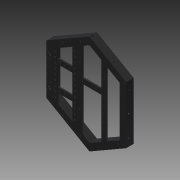
# Autodesk Inventor part: TSOP Array
Saved by Autodesk Inventor 2015 (Build 190159000, 159)
## iProperties
Created: 2016-02-25
Part Number: TSOP Array
Material: ABS Plastic
Document SubType Name: Modeling
Designer: James Yelland
Density: 1.06 g/cm^3
Appearance: Smooth - White
Mass: 118.644 g
Surface Area: 498.11 cm^2
Volume: 111.928 cm^3
Author: James Yelland
Autodesk Inventor part; units mm, degrees
ref_plane "YZ Plane" through (0, 0, 0) normal (1, 0, 0) x (0, 1, 0)
ref_plane "XZ Plane" through (0, 0, 0) normal (0, 1, 0) x (-1, 0, 0)
ref_plane "XY Plane" through (0, 0, 0) normal (0, 0, 1) x (1, 0, 0)
sketch "Sketch1" plane through (0, 0, 0) normal (0, 1, 0) x (-1, 0, 0)
  line L0 (0, 100) -> (86.6025, 50)
  line L1 (86.6025, 50) -> (86.6025, -50)
  line L2 (86.6025, -50) -> (0, -100)
  line L3 (0, 85) -> (73.6122, 42.5)
  line L4 (73.6122, 42.5) -> (73.6122, -42.5)
  line L5 (73.6122, -42.5) -> (0, -85)
  circle A0 centre (-69.3774, 54.1653) radius 1.6
  line L6 (-60.6222, 0) -> (-60.6222, -49.9998)
  line L7 (-60.6222, 0) -> (-60.6222, 49.9998)
  line L8 (0, -85) -> (-60.6222, -49.9998)
  line L9 (-60.6222, 49.9998) -> (0, 85)
  line L10 (-73.6122, -57.5) -> (-73.6122, 57.5)
  line L11 (0, 100) -> (-73.6122, 57.5)
  line L12 (-73.6122, -57.5) -> (0, -100)
  circle A1 centre (-69.3774, -54.1745) radius 1.6
  line L13 (-68.5014, -5.4) -> (-63.7014, -5.4)
  line L14 (-63.7014, -5.4) -> (-63.7014, 5.4)
  line L15 (-63.7014, 5.4) -> (-68.5014, 5.4)
  arc A2 (-68.5014, 2.5807) -> (-68.5014, -2.5807) centre (-67.5514, 0) ccw
  line L16 (-68.5014, -5.4) -> (-68.5014, -2.5807)
  line L17 (-68.5014, 2.5807) -> (-68.5014, 5.4)
  line L18 (-70.3014, 0) -> (-67.5514, 0)
  line L19 (-67.5514, 0) -> (-73.5514, 0)
  line L20 (-66.5387, -44.6515) -> (-62.3818, -42.2515)
  line L21 (-62.3818, -42.2515) -> (-67.7818, -32.8985)
  line L22 (-67.7818, -32.8985) -> (-71.9387, -35.2985)
  arc A3 (-70.5291, -37.7401) -> (-67.9484, -42.2099) centre (-68.416, -39.5) ccw
  line L23 (-66.5387, -44.6515) -> (-67.9484, -42.2099)
  line L24 (-70.5291, -37.7401) -> (-71.9387, -35.2985)
  line L25 (-70.7976, -40.875) -> (-68.416, -39.5)
  line L26 (-68.416, -39.5) -> (-73.6122, -42.5)
  line L27 (-36.0997, -73.3266) -> (-33.6997, -69.1696)
  line L28 (-33.6997, -69.1696) -> (-43.0528, -63.7696)
  line L29 (-43.0528, -63.7696) -> (-45.4528, -67.9266)
  arc A4 (-43.0112, -69.3362) -> (-38.5413, -71.9169) centre (-40.3013, -69.8038) ccw
  line L30 (-36.0997, -73.3266) -> (-38.5413, -71.9169)
  line L31 (-43.0112, -69.3362) -> (-45.4528, -67.9266)
  line L32 (-41.6763, -72.1854) -> (-40.3013, -69.8038)
  line L33 (-40.3013, -69.8038) -> (-43.3013, -75)
  line L34 (5.4, -94.95) -> (5.4, -90.15)
  line L35 (5.4, -90.15) -> (-5.4, -90.15)
  line L36 (-5.4, -90.15) -> (-5.4, -94.95)
  arc A5 (-2.5807, -94.95) -> (2.5807, -94.95) centre (0, -94) ccw
  line L37 (5.4, -94.95) -> (2.5807, -94.95)
  line L38 (-2.5807, -94.95) -> (-5.4, -94.95)
  line L39 (0, -96.75) -> (0, -94)
  line L40 (0, -94) -> (0, -100)
  line L41 (45.4528, -67.9266) -> (43.0528, -63.7696)
  line L42 (43.0528, -63.7696) -> (33.6997, -69.1696)
  line L43 (33.6997, -69.1696) -> (36.0997, -73.3266)
  arc A6 (38.5413, -71.9169) -> (43.0112, -69.3362) centre (40.3013, -69.8038) ccw
  line L44 (45.4528, -67.9266) -> (43.0112, -69.3362)
  line L45 (38.5413, -71.9169) -> (36.0997, -73.3266)
  line L46 (41.6763, -72.1854) -> (40.3013, -69.8038)
  line L47 (40.3013, -69.8038) -> (43.3013, -75)
  line L48 (84.9291, -42.7985) -> (80.7722, -40.3985)
  line L49 (80.7722, -40.3985) -> (75.3722, -49.7515)
  line L50 (75.3722, -49.7515) -> (79.5291, -52.1515)
  arc A7 (80.9388, -49.7099) -> (83.5195, -45.2401) centre (81.4064, -47) ccw
  line L51 (84.9291, -42.7985) -> (83.5195, -45.2401)
  line L52 (80.9388, -49.7099) -> (79.5291, -52.1515)
  line L53 (83.788, -48.375) -> (81.4064, -47)
  line L54 (81.4064, -47) -> (86.6025, -50)
  line L55 (81.5525, 5.4) -> (76.7525, 5.4)
  line L56 (76.7525, 5.4) -> (76.7525, -5.4)
  line L57 (76.7525, -5.4) -> (81.5525, -5.4)
  arc A8 (81.5525, -2.5807) -> (81.5525, 2.5807) centre (80.6025, 0) ccw
  line L58 (81.5525, 5.4) -> (81.5525, 2.5807)
  line L59 (81.5525, -2.5807) -> (81.5525, -5.4)
  line L60 (83.3525, 0) -> (80.6025, 0)
  line L61 (80.6025, 0) -> (86.6025, 0)
  line L62 (79.5291, 52.1515) -> (75.3722, 49.7515)
  line L63 (75.3722, 49.7515) -> (80.7722, 40.3985)
  line L64 (80.7722, 40.3985) -> (84.9291, 42.7985)
  arc A9 (83.5195, 45.2401) -> (80.9388, 49.7099) centre (81.4064, 47) ccw
  line L65 (79.5291, 52.1515) -> (80.9388, 49.7099)
  line L66 (83.5195, 45.2401) -> (84.9291, 42.7985)
  line L67 (83.788, 48.375) -> (81.4064, 47)
  line L68 (81.4064, 47) -> (86.6025, 50)
  line L69 (36.0997, 73.3266) -> (33.6997, 69.1696)
  line L70 (33.6997, 69.1696) -> (43.0528, 63.7696)
  line L71 (43.0528, 63.7696) -> (45.4528, 67.9266)
  arc A10 (43.0112, 69.3362) -> (38.5413, 71.9169) centre (40.3013, 69.8038) ccw
  line L72 (36.0997, 73.3266) -> (38.5413, 71.9169)
  line L73 (43.0112, 69.3362) -> (45.4528, 67.9266)
  line L74 (41.6763, 72.1854) -> (40.3013, 69.8038)
  line L75 (40.3013, 69.8038) -> (43.3013, 75)
  line L76 (-5.4, 94.95) -> (-5.4, 90.15)
  line L77 (-5.4, 90.15) -> (5.4, 90.15)
  line L78 (5.4, 90.15) -> (5.4, 94.95)
  arc A11 (2.5807, 94.95) -> (-2.5807, 94.95) centre (0, 94) ccw
  line L79 (-5.4, 94.95) -> (-2.5807, 94.95)
  line L80 (2.5807, 94.95) -> (5.4, 94.95)
  line L81 (0, 96.75) -> (0, 94)
  line L82 (0, 94) -> (0, 100)
  line L83 (-45.4528, 67.9266) -> (-43.0528, 63.7696)
  line L84 (-43.0528, 63.7696) -> (-33.6997, 69.1696)
  line L85 (-33.6997, 69.1696) -> (-36.0997, 73.3266)
  arc A12 (-38.5413, 71.9169) -> (-43.0112, 69.3362) centre (-40.3013, 69.8038) ccw
  line L86 (-45.4528, 67.9266) -> (-43.0112, 69.3362)
  line L87 (-38.5413, 71.9169) -> (-36.0997, 73.3266)
  line L88 (-41.6763, 72.1854) -> (-40.3013, 69.8038)
  line L89 (-40.3013, 69.8038) -> (-43.3013, 75)
  line L90 (-71.9387, 35.2985) -> (-67.7818, 32.8985)
  line L91 (-67.7818, 32.8985) -> (-62.3818, 42.2515)
  line L92 (-62.3818, 42.2515) -> (-66.5387, 44.6515)
  arc A13 (-67.9484, 42.2099) -> (-70.5291, 37.7401) centre (-68.416, 39.5) ccw
  line L93 (-71.9387, 35.2985) -> (-70.5291, 37.7401)
  line L94 (-67.9484, 42.2099) -> (-66.5387, 44.6515)
  line L95 (-70.7976, 40.875) -> (-68.416, 39.5)
  line L96 (-68.416, 39.5) -> (-73.6122, 42.5)
  dimension "d5" = 360
  dimension "d293" = 360
  dimension "d153" = 3.2
  dimension "d154" = 3.2
  dimension "d274" = 5.4
  dimension "d275" = 4.8
  dimension "d276" = 10.8
  dimension "d284" = 2.75
  dimension "d285" = 1.8
  dimension "d286" = 6
  constraints: 194 end point, 25 point on circle, 14 centre point, 1 point on line
  measures "d153" diameter of A1
  measures "d154" diameter of A0
  measures "d274" distance from line of L13 L18.end
  measures "d275" distance of L13.start L13.end
  measures "d276" distance of L13.end L14.end
  measures "d284" radius of A2
  measures "d285" horizontal distance of L18.start L13.start
  measures "d286" distance of L18.end L19.end
extrude "Extrusion1" add sketch "Sketch1" along normal blind 15 contours L0 L1 L2 L12 L10 L11 | A0 | A1
sketch "Sketch5" plane through (0, 15, 0) normal (0, 1, 0) x (1, 0, 0)
  circle A0 centre (-53.7917, 63.1699) radius 1.6
  circle A1 centre (-53.7917, -63.1699) radius 1.6
  line L0 (-73.6122, -42.5) -> (-73.6122, 42.5) projected
  line L1 (-73.6122, 42.5) -> (0, 85) projected
  line L2 (0, -85) -> (-73.6122, -42.5) projected
  line L3 (-86.6025, -50) -> (0, -100) projected
  line L4 (0, 100) -> (-86.6025, 50) projected
  line L5 (-86.6025, 50) -> (-86.6025, -50) projected
  circle A2 centre (69.3801, -54.1699) radius 1.6
  circle A3 centre (69.3801, 54.1699) radius 1.6
  line L6 (60.6222, -49.9998) -> (0, -85) projected
  line L7 (0, 85) -> (60.6222, 49.9998) projected
  line L8 (60.6222, 49.9998) -> (60.6222, -49.9998) projected
  line L9 (0, -100) -> (73.6122, -57.5) projected
  line L10 (73.6122, -57.5) -> (73.6122, 57.5) projected
  line L11 (73.6122, 57.5) -> (0, 100) projected
  point P0 (0, 0)
  dimension "d31" = 3.2
  dimension "d34" = 3.2
  dimension "d155" = 3.2
  dimension "d156" = 3.2
  constraints: 4 centre point
  measures "d31" diameter of A0
  measures "d34" diameter of A1
  measures "d155" diameter of A2
  measures "d156" diameter of A3
extrude "Extrusion5" cut sketch "Sketch5" against normal through all contours A0 | A1 | A2 | A3
sketch "Sketch6" plane through (0, 0, 0) normal (0, -1, 0) x (1, 0, 0)
  circle A0 centre (-29.6096, -40) radius 1.6
  circle A1 centre (-19.6096, 46.1471) radius 1.6
  circle A2 centre (28.6122, 39.8205) radius 1.6
  circle A3 centre (28.6122, -35.0619) radius 1.6
  circle A4 centre (13.3775, 15.699) radius 1.6
  circle A5 centre (-14.5314, 15.699) radius 1.6
  line L0 (-14.531, 20.699) -> (-14.6092, 20.699)
  line L1 (-14.6092, 20.699) -> (23.6131, 20.699)
  line L2 (23.6126, 10.699) -> (-14.6092, 10.699)
  line L3 (-73.6122, -42.5) -> (-63.6122, -48.2735)
  line L4 (-73.6122, -42.5) -> (-73.6122, 42.5)
  line L5 (-63.6122, 48.2735) -> (-73.6122, 42.5)
  circle A6 centre (-29.6096, 50) radius 1.6
  circle A7 centre (-29.6096, -50) radius 1.6
  line L6 (-63.6122, -20) -> (-34.6092, -20)
  line L7 (-63.6122, -30) -> (-34.6092, -30)
  line L8 (-63.6122, 20) -> (-34.6092, 20)
  line L9 (-34.6092, 30) -> (-63.6122, 30)
  line L10 (-63.6122, 30) -> (-63.6122, 48.2735)
  line L11 (-63.6122, -30) -> (-63.6122, -48.2735)
  line L12 (-34.6092, -20) -> (-34.6092, 20)
  circle A8 centre (-29.6096, -30) radius 1.6
  circle A9 centre (-29.6096, -20) radius 1.6
  circle A10 centre (-29.6096, -10) radius 1.6
  circle A11 centre (-29.6096, 0) radius 1.6
  circle A12 centre (-29.6096, 10) radius 1.6
  circle A13 centre (-29.6096, 20) radius 1.6
  circle A14 centre (-29.6096, 30) radius 1.6
  circle A15 centre (-29.6096, 40) radius 1.6
  circle A16 centre (-29.6096, 60) radius 1.6
  circle A17 centre (-29.6096, -60) radius 1.6
  circle A18 centre (-39.1109, 25) radius 1.6
  circle A19 centre (-49.1109, 25) radius 1.6
  circle A20 centre (-59.1109, 25) radius 1.6
  circle A21 centre (-39.1109, -25) radius 1.6
  circle A22 centre (-49.1109, -25) radius 1.6
  circle A23 centre (-59.1109, -25) radius 1.6
  circle A24 centre (-68.6122, -40) radius 1.6
  circle A25 centre (-68.6122, -30) radius 1.6
  circle A26 centre (-68.6122, -20) radius 1.6
  circle A27 centre (-68.6122, -10) radius 1.6
  circle A28 centre (-68.6122, 0) radius 1.6
  circle A29 centre (-68.6122, 10) radius 1.6
  circle A30 centre (-68.6122, 20) radius 1.6
  circle A31 centre (-68.6122, 30) radius 1.6
  circle A32 centre (-68.6122, 40) radius 1.6
  circle A33 centre (-19.6096, -36.3314) radius 1.6
  line L13 (-19.6096, 10) -> (-29.6096, 10)
  line L14 (23.6126, -71.3672) -> (33.6126, -65.5937)
  line L15 (23.6131, 71.367) -> (33.6126, 65.5937)
  line L16 (-34.6092, 65.0184) -> (-14.6092, 76.5654)
  line L17 (-14.6092, 10.699) -> (-14.6092, -76.5654)
  line L18 (-14.6092, -76.5654) -> (-34.6092, -65.0184)
  line L19 (-14.6092, 20.699) -> (-14.6092, 76.5654)
  line L20 (23.6131, 20.699) -> (23.6131, 71.367)
  line L21 (23.6126, -71.3672) -> (23.6126, 10.699)
  line L22 (33.6126, -65.5937) -> (33.6126, 65.5937)
  line L23 (-34.6092, 30) -> (-34.6092, 65.0184)
  line L24 (-34.6092, -65.0184) -> (-34.6092, -30)
  line L25 (-63.6122, -20) -> (-63.6122, 20)
  line L26 (-73.6122, -42.5) -> (-73.6122, 42.5)
  point P0 (0, -13.7917)
  dimension "d168" = 3.2
  dimension "d169" = 3.2
  dimension "d170" = 3.2
  dimension "d171" = 3.2
  dimension "d209" = 3.2
  dimension "d222" = 10
  constraints: 54 end point, 34 centre point, 12 vertical, 1 collinear, 1 horizontal, 1 point on line
  measures "d168" diameter of A5
  measures "d169" diameter of A4
  measures "d170" diameter of A2
  measures "d171" diameter of A3
  measures "d209" diameter of A33
  measures "d222" distance of L13.start L13.end
extrude "Extrusion6" add sketch "Sketch6" against normal blind 3
sketch "Sketch7" plane through (0, 15, 0) normal (0, 1, 0) x (1, 0, 0)
  circle A0 centre (69.3801, 54.1699) radius 1.6 projected
  circle A1 centre (-53.7917, 63.1699) radius 1.6 projected
  circle A2 centre (-53.7917, -63.1699) radius 1.6 projected
  circle A3 centre (69.3801, -54.1699) radius 1.6 projected
  line L0 (-73.6122, -42.5) -> (-73.6122, 42.5) projected
  line L1 (-73.6122, 42.5) -> (0, 85) projected
  line L2 (0, -85) -> (-73.6122, -42.5) projected
  line L3 (-86.6025, -50) -> (0, -100) projected
  line L4 (0, 100) -> (-86.6025, 50) projected
  line L5 (-86.6025, 50) -> (-86.6025, -50) projected
  circle A4 centre (-80.1075, -20) radius 1.6
  circle A5 centre (-80.1075, 20) radius 1.6
  line L6 (60.6222, -49.9998) -> (0, -85) projected
  line L7 (0, 85) -> (60.6222, 49.9998) projected
  line L8 (60.6222, 49.9998) -> (60.6222, -49.9998) projected
  line L9 (0, -100) -> (73.6122, -57.5) projected
  line L10 (73.6122, -57.5) -> (73.6122, 57.5) projected
  line L11 (73.6122, 57.5) -> (0, 100) projected
  line L12 (0, 100) -> (73.6122, 57.5) projected
  circle A6 centre (-18.3996, -81.8767) radius 1.6
  circle A7 centre (57.3685, -59.3781) radius 1.6
  line L13 (73.6122, -57.5) -> (73.6122, 57.5) projected
  circle A8 centre (-18.4029, 81.8748) radius 1.6
  circle A9 centre (57.3685, 59.3781) radius 1.6
  line L14 (0, 100) -> (-86.6025, 50) projected
  line L15 (-15.1376, -76.2603) -> (-18.3996, -81.8767)
  line L16 (-73.6122, 42.5) -> (0, 85) projected
  line L17 (-15.1554, 76.25) -> (-18.4029, 81.8748)
  line L18 (0, 85) -> (60.6222, 49.9998) projected
  line L19 (54.121, 53.7532) -> (57.3685, 59.3781)
  line L20 (54.121, -53.7532) -> (57.3685, -59.3781)
  point P0 (0, 0)
  dimension "d135" = 6.495
  dimension "d136" = 6.495
  dimension "d138" = 6.495
  dimension "d139" = 6.495
  dimension "d157" = 3.2
  dimension "d158" = 3.2
  dimension "d159" = 3.2
  dimension "d160" = 3.2
  dimension "d161" = 3.2
  dimension "d162" = 3.2
  constraints: 8 end point, 6 centre point, 4 point on line
  measures "d135" distance of L15.start L15.end
  measures "d136" distance of L17.start L17.end
  measures "d138" distance of L19.start L19.end
  measures "d139" distance of L20.start L20.end
  measures "d157" diameter of A6
  measures "d158" diameter of A4
  measures "d159" diameter of A5
  measures "d160" diameter of A8
  measures "d161" diameter of A9
  measures "d162" diameter of A7
extrude "Extrusion7" cut sketch "Sketch7" against normal through all contours A4 | A5 | A6 | A7 | A8 | A9
sketch "Sketch10" plane through (0, 15, 0) normal (0, 1, 0) x (1, 0, 0)
  circle A0 centre (69.3801, 54.1699) radius 1.6 projected
  circle A1 centre (-53.7917, 63.1699) radius 1.6 projected
  circle A2 centre (-53.7917, -63.1699) radius 1.6 projected
  circle A3 centre (69.3801, -54.1699) radius 1.6 projected
  line L0 (60.6222, -49.9998) -> (0, -85) projected
  line L1 (0, -85) -> (-73.6122, -42.5) projected
  line L2 (-73.6122, -42.5) -> (-73.6122, 42.5) projected
  line L3 (-73.6122, 42.5) -> (0, 85) projected
  line L4 (0, 85) -> (60.6222, 49.9998) projected
  line L5 (60.6222, 49.9998) -> (60.6222, -49.9998) projected
  line L6 (0, -100) -> (73.6122, -57.5) projected
  line L7 (73.6122, -57.5) -> (73.6122, 57.5) projected
  line L8 (73.6122, 57.5) -> (0, 100) projected
  line L9 (0, 100) -> (-86.6025, 50) projected
  line L10 (-86.6025, 50) -> (-86.6025, -50) projected
  line L11 (-86.6025, -50) -> (0, -100) projected
  circle A4 centre (-80.1075, 30) radius 3
  circle A5 centre (-80.1075, -30) radius 3
  point P0 (0, 0)
  dimension "d142" = 6
  dimension "d144" = 6
  constraints: 2 centre point
  measures "d142" diameter of A4
  measures "d144" diameter of A5
extrude "Extrusion10" cut sketch "Sketch10" against normal through all contours A4 | A5
sketch "Sketch13" plane through (60.6222, 0, 49.9998) normal (-1, 0, 0) x (0, 0, 1)
  circle A0 centre (-71.9998, 3) radius 1.4
  circle A1 centre (-27.9998, 3) radius 1.4
  circle A2 centre (-39.5858, 3.175) radius 1.4
  circle A3 centre (-60.4138, 3.175) radius 1.4
  dimension "d213" = 2.8
  dimension "d217" = 2.8
  dimension "d218" = 2.8
  constraints: 4 centre point
  measures "d213" diameter of A0
  measures "d217" diameter of A2
  measures "d218" diameter of A3
extrude "Extrusion12" cut sketch "Sketch13" against normal blind 10
sketch "Sketch20" plane through (0, 0, 0) normal (0, -1, 0) x (1, 0, 0)
  circle A0 centre (-80.1075, -30) radius 3 projected
  circle A1 centre (-80.1075, 30) radius 3 projected
  circle A2 centre (-18.4029, -81.8748) radius 1.6 projected
  circle A3 centre (-18.3996, 81.8767) radius 1.6 projected
  circle A4 centre (-80.1075, -20) radius 1.6 projected
  circle A5 centre (-80.1075, 20) radius 1.6 projected
  circle A6 centre (57.3685, 59.3781) radius 1.6 projected
  circle A7 centre (57.3685, -59.3781) radius 1.6 projected
  line L0 (-14.6092, 76.5654) -> (0, 85) projected
  line L1 (0, 85) -> (23.6131, 71.367) projected
  line L2 (23.6131, 71.367) -> (23.6131, 20.699) projected
  line L3 (23.6131, 20.699) -> (-14.6092, 20.699) projected
  line L4 (-14.6092, 20.699) -> (-14.6092, 76.5654) projected
  line L5 (-34.6092, 65.0184) -> (-34.6092, 30) projected
  line L6 (-34.6092, 30) -> (-63.6122, 30) projected
  line L7 (-63.6122, 30) -> (-63.6122, 48.2735) projected
  line L8 (-63.6122, 48.2735) -> (-34.6092, 65.0184) projected
  line L9 (-63.6122, -48.2735) -> (-63.6122, -30) projected
  line L10 (-63.6122, -30) -> (-34.6092, -30) projected
  line L11 (-34.6092, -30) -> (-34.6092, -65.0184) projected
  line L12 (-34.6092, -65.0184) -> (-63.6122, -48.2735) projected
  line L13 (-14.6092, -76.5654) -> (-14.6092, 10.699) projected
  line L14 (-14.6092, 10.699) -> (23.6126, 10.699) projected
  line L15 (23.6126, 10.699) -> (23.6126, -71.3672) projected
  line L16 (23.6126, -71.3672) -> (0, -85) projected
  line L17 (0, -85) -> (-14.6092, -76.5654) projected
  circle A8 centre (28.6122, -35.0619) radius 1.6 projected
  circle A9 centre (-29.6096, -40) radius 1.6 projected
  circle A10 centre (13.3775, 15.699) radius 1.6 projected
  circle A11 centre (-14.5314, 15.699) radius 1.6 projected
  circle A12 centre (28.6122, 39.8205) radius 1.6 projected
  circle A13 centre (-19.6096, 46.1471) radius 1.6 projected
  circle A14 centre (-29.6096, 50) radius 1.6 projected
  circle A15 centre (-29.6096, -50) radius 1.6 projected
  circle A16 centre (-29.6096, -30) radius 1.6 projected
  circle A17 centre (-29.6096, -20) radius 1.6 projected
  circle A18 centre (-29.6096, -10) radius 1.6 projected
  circle A19 centre (-29.6096, 0) radius 1.6 projected
  circle A20 centre (-29.6096, 10) radius 1.6 projected
  circle A21 centre (-29.6096, 20) radius 1.6 projected
  circle A22 centre (-29.6096, 30) radius 1.6 projected
  circle A23 centre (-29.6096, 40) radius 1.6 projected
  circle A24 centre (-29.6096, 60) radius 1.6 projected
  circle A25 centre (-29.6096, -60) radius 1.6 projected
  circle A26 centre (-39.1109, 25) radius 1.6 projected
  circle A27 centre (-49.1109, 25) radius 1.6 projected
  circle A28 centre (-59.1109, 25) radius 1.6 projected
  circle A29 centre (-49.1109, -25) radius 1.6 projected
  circle A30 centre (-59.1109, -25) radius 1.6 projected
  circle A31 centre (-39.1109, -25) radius 1.6 projected
  circle A32 centre (-68.6122, -40) radius 1.6 projected
  circle A33 centre (-68.6122, -30) radius 1.6 projected
  circle A34 centre (-68.6122, 20) radius 1.6 projected
  circle A35 centre (-68.6122, 10) radius 1.6 projected
  circle A36 centre (-68.6122, 0) radius 1.6 projected
  circle A37 centre (-68.6122, -10) radius 1.6 projected
  circle A38 centre (-68.6122, -20) radius 1.6 projected
  circle A39 centre (-68.6122, 30) radius 1.6 projected
  circle A40 centre (-68.6122, 40) radius 1.6 projected
  circle A41 centre (-19.6096, -36.3314) radius 1.6 projected
  line L18 (-34.6092, 20) -> (-34.6092, -20) projected
  line L19 (-34.6092, -20) -> (-63.6122, -20) projected
  line L20 (-63.6122, -20) -> (-63.6122, 20) projected
  line L21 (-63.6122, 20) -> (-34.6092, 20) projected
  circle A42 centre (69.3801, -54.1699) radius 1.6 projected
  circle A43 centre (-53.7917, -63.1699) radius 1.6 projected
  circle A44 centre (-53.7917, 63.1699) radius 1.6 projected
  circle A45 centre (69.3801, 54.1699) radius 1.6 projected
  line L22 (33.6126, -65.5937) -> (33.6126, 65.5937) projected
  line L23 (33.6126, 65.5937) -> (60.6222, 49.9998) projected
  line L24 (60.6222, 49.9998) -> (60.6222, -49.9998) projected
  line L25 (60.6222, -49.9998) -> (33.6126, -65.5937) projected
  line L26 (70.5291, 37.7401) -> (71.9387, 35.2985) projected
  line L27 (71.9387, 35.2985) -> (67.7818, 32.8985) projected
  line L28 (67.7818, 32.8985) -> (62.3818, 42.2515) projected
  line L29 (62.3818, 42.2515) -> (66.5387, 44.6515) projected
  line L30 (66.5387, 44.6515) -> (67.9484, 42.2099) projected
  arc A46 (70.5291, 37.7401) -> (67.9484, 42.2099) centre (68.416, 39.5) ccw projected
  line L31 (43.0112, 69.3362) -> (45.4528, 67.9266) projected
  line L32 (45.4528, 67.9266) -> (43.0528, 63.7696) projected
  line L33 (43.0528, 63.7696) -> (33.6997, 69.1696) projected
  line L34 (33.6997, 69.1696) -> (36.0997, 73.3266) projected
  line L35 (36.0997, 73.3266) -> (38.5413, 71.9169) projected
  arc A47 (43.0112, 69.3362) -> (38.5413, 71.9169) centre (40.3013, 69.8038) ccw projected
  line L36 (2.5807, 94.95) -> (5.4, 94.95) projected
  line L37 (5.4, 94.95) -> (5.4, 90.15) projected
  line L38 (5.4, 90.15) -> (-5.4, 90.15) projected
  line L39 (-5.4, 90.15) -> (-5.4, 94.95) projected
  line L40 (-5.4, 94.95) -> (-2.5807, 94.95) projected
  arc A48 (2.5807, 94.95) -> (-2.5807, 94.95) centre (0, 94) ccw projected
  line L41 (-38.5413, 71.9169) -> (-36.0997, 73.3266) projected
  line L42 (-36.0997, 73.3266) -> (-33.6997, 69.1696) projected
  line L43 (-33.6997, 69.1696) -> (-43.0528, 63.7696) projected
  line L44 (-43.0528, 63.7696) -> (-45.4528, 67.9266) projected
  line L45 (-45.4528, 67.9266) -> (-43.0112, 69.3362) projected
  arc A49 (-38.5413, 71.9169) -> (-43.0112, 69.3362) centre (-40.3013, 69.8038) ccw projected
  line L46 (-80.9388, 49.7099) -> (-79.5291, 52.1515) projected
  line L47 (-79.5291, 52.1515) -> (-75.3722, 49.7515) projected
  line L48 (-75.3722, 49.7515) -> (-80.7722, 40.3985) projected
  line L49 (-80.7722, 40.3985) -> (-84.9291, 42.7985) projected
  line L50 (-84.9291, 42.7985) -> (-83.5195, 45.2401) projected
  arc A50 (-80.9388, 49.7099) -> (-83.5195, 45.2401) centre (-81.4064, 47) ccw projected
  line L51 (-81.5525, 2.5807) -> (-81.5525, 5.4) projected
  line L52 (-81.5525, 5.4) -> (-76.7525, 5.4) projected
  line L53 (-76.7525, 5.4) -> (-76.7525, -5.4) projected
  line L54 (-76.7525, -5.4) -> (-81.5525, -5.4) projected
  line L55 (-81.5525, -5.4) -> (-81.5525, -2.5807) projected
  arc A51 (-81.5525, 2.5807) -> (-81.5525, -2.5807) centre (-80.6025, 0) ccw projected
  line L56 (-83.5195, -45.2401) -> (-84.9291, -42.7985) projected
  line L57 (-84.9291, -42.7985) -> (-80.7722, -40.3985) projected
  line L58 (-80.7722, -40.3985) -> (-75.3722, -49.7515) projected
  line L59 (-75.3722, -49.7515) -> (-79.5291, -52.1515) projected
  line L60 (-79.5291, -52.1515) -> (-80.9388, -49.7099) projected
  arc A52 (-83.5195, -45.2401) -> (-80.9388, -49.7099) centre (-81.4064, -47) ccw projected
  line L61 (-43.0112, -69.3362) -> (-45.4528, -67.9266) projected
  line L62 (-45.4528, -67.9266) -> (-43.0528, -63.7696) projected
  line L63 (-43.0528, -63.7696) -> (-33.6997, -69.1696) projected
  line L64 (-33.6997, -69.1696) -> (-36.0997, -73.3266) projected
  line L65 (-36.0997, -73.3266) -> (-38.5413, -71.9169) projected
  arc A53 (-43.0112, -69.3362) -> (-38.5413, -71.9169) centre (-40.3013, -69.8038) ccw projected
  line L66 (-2.5807, -94.95) -> (-5.4, -94.95) projected
  line L67 (-5.4, -94.95) -> (-5.4, -90.15) projected
  line L68 (-5.4, -90.15) -> (5.4, -90.15) projected
  line L69 (5.4, -90.15) -> (5.4, -94.95) projected
  line L70 (5.4, -94.95) -> (2.5807, -94.95) projected
  arc A54 (-2.5807, -94.95) -> (2.5807, -94.95) centre (0, -94) ccw projected
  line L71 (38.5413, -71.9169) -> (36.0997, -73.3266) projected
  line L72 (36.0997, -73.3266) -> (33.6997, -69.1696) projected
  line L73 (33.6997, -69.1696) -> (43.0528, -63.7696) projected
  line L74 (43.0528, -63.7696) -> (45.4528, -67.9266) projected
  line L75 (45.4528, -67.9266) -> (43.0112, -69.3362) projected
  arc A55 (38.5413, -71.9169) -> (43.0112, -69.3362) centre (40.3013, -69.8038) ccw projected
  line L76 (67.9484, -42.2099) -> (66.5387, -44.6515) projected
  line L77 (66.5387, -44.6515) -> (62.3818, -42.2515) projected
  line L78 (62.3818, -42.2515) -> (67.7818, -32.8985) projected
  line L79 (67.7818, -32.8985) -> (71.9387, -35.2985) projected
  line L80 (71.9387, -35.2985) -> (70.5291, -37.7401) projected
  arc A56 (67.9484, -42.2099) -> (70.5291, -37.7401) centre (68.416, -39.5) ccw projected
  line L81 (68.5014, -2.5807) -> (68.5014, -5.4) projected
  line L82 (68.5014, -5.4) -> (63.7014, -5.4) projected
  line L83 (63.7014, -5.4) -> (63.7014, 5.4) projected
  line L84 (63.7014, 5.4) -> (68.5014, 5.4) projected
  line L85 (68.5014, 5.4) -> (68.5014, 2.5807) projected
  arc A57 (68.5014, -2.5807) -> (68.5014, 2.5807) centre (67.5514, 0) ccw projected
  line L86 (0, 100) -> (-86.6025, 50) projected
  line L87 (-86.6025, 50) -> (-86.6025, -50) projected
  line L88 (-86.6025, -50) -> (0, -100) projected
  line L89 (0, -100) -> (73.6122, -57.5) projected
  line L90 (73.6122, -57.5) -> (73.6122, 57.5) projected
  line L91 (73.6122, 57.5) -> (0, 100) projected
  point P0 (0, 0)
extrude "Extrusion18" add sketch "Sketch20" against normal blind 2 contours L26 L27 L28 L29 L30 A46 | L31 L32 L33 L34 L35 A47 | L36 L37 L38 L39 L40 A48 | L41 L42 L43 L44 L45 A49 | L46 L47 L48 L49 L50 A50 | L51 L52 L53 L54 L55 A51 | L56 L57 L58 L59 L60 A52 | L61 L62 L63 L64 L65 A53 | L66 L67 L68 L69 L70 A54 | L71 L72 L73 L74 L75 A55 | L76 L77 L78 L79 L80 A56 | L81 L82 L83 L84 L85 A57
sketch "Sketch21" plane through (63.7014, 15, 5.4) normal (1, 0, 0) x (0, 0, -1)
  line L0 (0, 0) -> (10.8, 0) projected
  line L1 (5.4, 0) -> (5.4, -9.5)
  circle A0 centre (5.4, -9.5) radius 1.75
  point P0 (5.4, -15)
  dimension "d297" = 9.5
  dimension "d298" = 3.5
  constraints: 2 end point, 1 centre point, 1 coincident, 1 midpoint, 1 vertical
  measures "d297" distance of L1.start L1.end
  measures "d298" diameter of A0
extrude "Extrusion19" cut sketch "Sketch21" along normal through all
sketch "Sketch22" plane through (62.3818, 2, -42.2515) normal (0.8660254, 0, -0.5) x (-0.5, 0, -0.8660254)
  line L0 (-10.8, 13) -> (0, 13) projected
  line L1 (-5.4, 13) -> (-5.4, 3.5)
  circle A0 centre (-5.4, 3.5) radius 1.75
  point P0 (-5.4, -2)
  dimension "d301" = 9.5
  dimension "d302" = 3.5
  constraints: 2 end point, 1 centre point, 1 coincident, 1 midpoint, 1 vertical
  measures "d301" distance of L1.start L1.end
  measures "d302" diameter of A0
extrude "Extrusion20" cut sketch "Sketch22" along normal through all
sketch "Sketch23" plane through (67.7818, 2, 32.8985) normal (0.8660254, 0, 0.5) x (0.5, 0, -0.8660254)
  line L0 (-10.8, 13) -> (0, 13) projected
  line L1 (-5.4, 13) -> (-5.4, 3.5)
  circle A0 centre (-5.4, 3.5) radius 1.75
  point P0 (-5.4, -2)
  dimension "d305" = 9.5
  dimension "d306" = 3.5
  constraints: 2 end point, 1 centre point, 1 coincident, 1 midpoint, 1 vertical
  measures "d305" distance of L1.start L1.end
  measures "d306" diameter of A0
extrude "Extrusion21" cut sketch "Sketch23" along normal through all
sketch "Sketch24" plane through (33.6997, 2, -69.1696) normal (0.5, 0, -0.8660254) x (-0.8660254, 0, -0.5)
  line L0 (-10.8, 13) -> (0, 13) projected
  line L1 (-5.4, 13) -> (-5.4, 3.5)
  circle A0 centre (-5.4, 3.5) radius 1.75
  point P0 (-5.4, -2)
  dimension "d309" = 9.5
  dimension "d310" = 3.5
  constraints: 2 end point, 1 centre point, 1 coincident, 1 midpoint, 1 vertical
  measures "d309" distance of L1.start L1.end
  measures "d310" diameter of A0
extrude "Extrusion22" cut sketch "Sketch24" along normal through all
sketch "Sketch25" plane through (5.4, 15, -90.15) normal (0, 0, -1) x (-1, 0, 0)
  line L0 (0, 0) -> (10.8, 0) projected
  line L1 (5.4, 0) -> (5.4, -9.5)
  line L2 (5.4, -15) -> (5.4, 0) projected
  circle A0 centre (5.4, -9.5) radius 1.75
  dimension "d313" = 9.5
  dimension "d314" = 3.5
  constraints: 2 end point, 1 centre point, 1 coincident, 1 midpoint, 1 point on line
  measures "d313" distance of L1.start L1.end
  measures "d314" diameter of A0
extrude "Extrusion23" cut sketch "Sketch25" along normal through all
pattern_circular "Circular Pattern6" count 5 over 240 about axis through (0, -10, 0) along (0, 1, 0) of "Extrusion22"
pattern_circular "Circular Pattern7" count 4 over 180 about axis through (0, -10, 0) along (0, 1, 0) of "Extrusion23"
body "Solid1"
